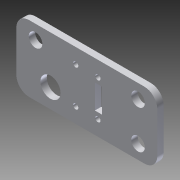
# Autodesk Inventor part: V5 Shooter Bearing Encoder Plate
Saved by Autodesk Inventor 2014 SP1 (Build 180222100, 222)
## iProperties
Created: 2012-02-08
Part Number: V5 Shooter Bearing Encoder Plate
Material: Polycarbonate, Clear
Document SubType Name: Modeling
Designer: Moses
Mass: 7.70573 g
Surface Area: 51.6769 cm^2
Volume: 6.42144 cm^3
Density: 1.2 g/cm^3
Appearance: Smooth - White
Author: Moses
Autodesk Inventor part; units mm, degrees
ref_plane "YZ Plane" through (0, 0, 0) normal (1, 0, 0) x (0, 1, 0)
ref_plane "XZ Plane" through (0, 0, 0) normal (0, 1, 0) x (-1, 0, 0)
ref_plane "XY Plane" through (0, 0, 0) normal (0, 0, 1) x (1, 0, 0)
sketch "Sketch1" plane through (0, 0, 0) normal (0, 0, 1) x (1, 0, 0)
  circle A0 centre (-194.945, 6.4301) radius 3.3782
  circle A1 centre (-194.945, 25.4801) radius 3.3782
  circle A2 centre (-144.145, 6.4301) radius 3.3782
  circle A3 centre (-144.145, 25.4801) radius 3.3782
  circle A4 centre (-169.545, 15.9551) radius 14.2875
  line L0 (-254, -1.8249) -> (254, -1.8249) construction
  line L1 (-247.65, 40.5304) -> (247.65, 40.5304) construction
  line L2 (-204.47, -0.5549) -> (-204.47, 32.4651)
  line L3 (-204.47, 32.4651) -> (-134.62, 32.4651)
  line L4 (-134.62, 32.4651) -> (-134.62, -0.5549)
  line L5 (-134.62, -0.5549) -> (-204.47, -0.5549)
  point P0 (0, 0)
extrude "Extrusion1" add sketch "Sketch1" along normal blind 3.175 contours A0 | A4 | L2 L3 L4 L5
fillet "Fillet1" radius 6.35 4 edges at (-204.47, 32.4651, 1.5875) (-204.47, -0.5549, 1.5875) (-134.62, 32.4651, 1.5875) (-134.62, -0.5549, 1.5875)
sketch "Sketch2" plane through (0, 0, 3.175) normal (0, 0, 1) x (1, 0, 0)
  line L0 (-134.62, 26.1151) -> (-134.62, 5.7951) projected
  line L1 (-198.12, 32.4651) -> (-140.97, 32.4651) projected
  line L2 (-204.47, 5.7951) -> (-204.47, 26.1151) projected
  line L3 (-140.97, -0.5549) -> (-198.12, -0.5549) projected
  line L4 (-169.545, 32.4651) -> (-169.545, -0.5549) construction
  line L5 (-204.47, 15.9551) -> (-134.62, 15.9551) construction
  circle A0 centre (-175.045, 24.9551) radius 1.3
  circle A1 centre (-164.045, 24.9551) radius 1.3
  circle A2 centre (-175.045, 6.9551) radius 1.3
  circle A3 centre (-164.045, 6.9551) radius 1.3
  line L6 (-175.045, 24.9551) -> (-164.045, 24.9551) construction
  line L7 (-175.045, 6.9551) -> (-164.045, 6.9551) construction
  line L8 (-175.045, 24.9551) -> (-175.045, 6.9551) construction
  line L9 (-165.545, 21.9551) -> (-165.545, 9.9551)
  line L10 (-165.545, 9.9551) -> (-162.045, 9.9551)
  line L11 (-162.045, 9.9551) -> (-162.045, 21.9551)
  line L12 (-162.045, 21.9551) -> (-165.545, 21.9551)
  circle A4 centre (-187.545, 8.9551) radius 5
  point P0 (0, 0)
  point P1 (-169.545, 6.9551)
  point P2 (-175.045, 15.9551)
  point P3 (-162.045, 15.9551)
  dimension "d7" = 2.6
  dimension "d10" = 11
  dimension "d13" = 18
  dimension "d16" = 12
  dimension "d17" = 3.5
  dimension "d18" = 4
  dimension "d19" = 10
  dimension "d20" = 7
  dimension "d21" = 18
  constraints: 18 end point, 7 midpoint, 5 centre point, 4 parallel, 3 perpendicular, 3 point on line, 1 horizontal, 1 vertical, 6 other
  measures "d7" diameter of A0
  measures "d10" distance of L6.start L6.end
  measures "d13" distance of L6.start L7.start
  measures "d16" distance of L9.start L9.end
  measures "d17" distance of L9.end L10.end
  measures "d18" distance between parallel lines of L9 L4
  measures "d19" diameter of A4
  measures "d20" distance from line of L5 A4.centre
  measures "d21" distance from line of L4 A4.centre
extrude "Extrusion2" cut sketch "Sketch2" against normal through all
equation "\"d2\" = d1"
equation "\"d1\" = 9.525"
body "Solid1"
